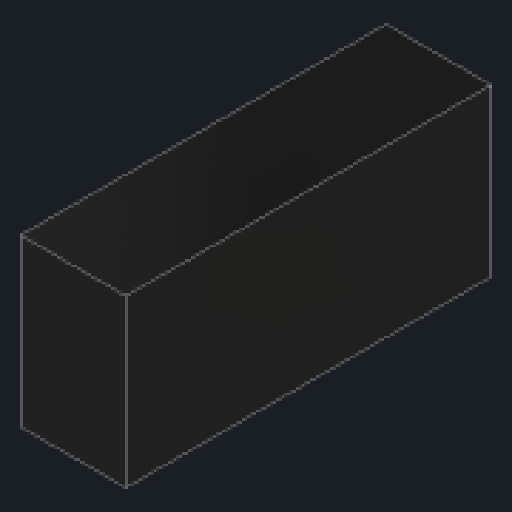
# Autodesk Inventor part: lipo3s650
Saved by Autodesk Inventor 2023 (Build 270158000, 158)
## iProperties
Created: 2024-04-13
Part Number: lipo3s650
Material: Acetal Resin, Black
Document SubType Name: Modeling
Designer: szymo
Density: 1.425 g/cm^3
Appearance: Smooth - Black
Mass: 65 g
Surface Area: 78.86 cm^2
Volume: 40.26 cm^3
Author: szymo
Autodesk Inventor part; units mm, degrees
ref_plane "YZ Plane" through (0, 0, 0) normal (1, 0, 0) x (0, 1, 0)
ref_plane "XZ Plane" through (0, 0, 0) normal (0, 1, 0) x (-1, 0, 0)
ref_plane "XY Plane" through (0, 0, 0) normal (0, 0, 1) x (1, 0, 0)
sketch "Sketch2" plane through (0, 0, 0) normal (0, 1, 0) x (-1, 0, 0)
  line L0 (0, 0) -> (-18, 0)
  line L1 (-18, 0) -> (-18, -66)
  line L2 (-18, -66) -> (0, -66)
  line L3 (0, -66) -> (0, 0)
  dimension "d0" = 18
  dimension "d1" = 66
  constraints: 8 end point, 2 parallel, 1 horizontal, 1 perpendicular
  measures "d0" distance of L2.end L1.end
  measures "d1" distance of L1.end L0.end
extrude "Extrusion1" add sketch "Sketch2" along normal blind 30
body "Solid1"
